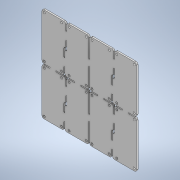
# Autodesk Inventor part: Part1
Saved by Autodesk Inventor 2021 (Build 250183000, 183)
## iProperties
Created: 2021-05-25
Part Number: Part1
Material: 一般
Document SubType Name: Modeling
Designer: admin
Density: 1 g/cm^3
Appearance: 既定
Author: admin
Autodesk Inventor part; units mm, degrees
ref_plane "YZ Plane" through (0, 0, 0) normal (1, 0, 0) x (0, 1, 0)
ref_plane "XZ Plane" through (0, 0, 0) normal (0, 1, 0) x (-1, 0, 0)
ref_plane "XY Plane" through (0, 0, 0) normal (0, 0, 1) x (1, 0, 0)
sketch "スケッチ1" plane through (0, 0, 0) normal (0, 0, 1) x (1, 0, 0)
  line L0 (0, 0) -> (49.5, 0)
  line L1 (49.5, 0) -> (49.5, 49.5)
  line L2 (49.5, 49.5) -> (0, 49.5)
  line L3 (0, 49.5) -> (0, 0)
  dimension "d0" = 49.5
  dimension "d1" = 49.5
  constraints: 8 end point, 2 parallel, 1 horizontal, 1 perpendicular
  measures "d0" distance of L2.end L1.end
  measures "d1" distance of L1.end L0.end
extrude "押し出し1" add sketch "スケッチ1" along normal blind 1.6
sketch "スケッチ2" plane through (0, 0, 1.6) normal (0, 0, 1) x (1, 0, 0)
  line L0 (0, 0) -> (49.5, 0) projected
  line L1 (24.75, 0) -> (24.75, 49.5) construction
  line L2 (49.5, 49.5) -> (0, 49.5) projected
  line L3 (49.5, 0) -> (49.5, 49.5) projected
  line L4 (49.5, 24.75) -> (0, 24.75) construction
  line L5 (0, 49.5) -> (0, 0) projected
  arc A0 (24.75, 23.25) -> (26.25, 24.75) centre (24.75, 24.75) ccw
  line L6 (26.25, 49.5) -> (26.25, 33.125) construction
  line L7 (23.25, 24.75) -> (23.25, 16.375)
  arc A1 (24.75, 26.25) -> (23.25, 24.75) centre (24.75, 24.75) ccw
  line L8 (24.75, 23.25) -> (24.25, 23.25)
  line L9 (24.75, 26.25) -> (25.25, 26.25)
  line L10 (24.25, 23.25) -> (24.25, 16.375)
  line L11 (25.25, 49.5) -> (25.25, 33.125) construction
  line L12 (23.25, 16.375) -> (24.25, 16.375)
  line L13 (24.25, 16.375) -> (24.25, 8.375) construction
  line L14 (24.25, 8.375) -> (23.25, 8.375) construction
  line L15 (23.25, 8.375) -> (23.25, 16.375) construction
  line L16 (25.25, 41.125) -> (26.25, 41.125) construction
  line L17 (26.25, 41.125) -> (26.25, 33.125) construction
  line L18 (26.25, 33.125) -> (25.25, 33.125)
  line L19 (25.25, 33.125) -> (25.25, 41.125) construction
  line L20 (21.3132, 37.125) -> (36.5279, 37.125) construction
  line L21 (13.313, 12.375) -> (31.136, 12.375) construction
  line L22 (23.25, 16.375) -> (23.25, 0) construction
  line L23 (24.25, 16.375) -> (24.25, 0.75) construction
  line L24 (25.25, 33.125) -> (25.25, 26.25)
  line L25 (26.25, 33.125) -> (26.25, 24.75)
  line L26 (25.25, 49.5) -> (26.25, 49.5)
  line L27 (26.25, 49.5) -> (26.25, 41.125)
  line L28 (26.25, 41.125) -> (25.25, 41.125)
  line L29 (25.25, 41.125) -> (25.25, 49.5)
  line L30 (23.25, 8.375) -> (24.25, 8.375)
  line L31 (24.25, 8.375) -> (24.25, 0)
  line L32 (24.25, 0) -> (23.25, 0)
  line L33 (23.25, 0) -> (23.25, 8.375)
  point P0 (25.25, 0)
  point P1 (25.25, 49.5)
  point P2 (25.25, 37.125)
  point P3 (24.25, 12.375)
  point P4 (25.25, 37.125)
  point P5 (24.25, 0)
  dimension "d31" = 3
  dimension "d32" = 1
  dimension "d33" = 8
  dimension "d34" = 24.75
  dimension "d35" = 49.5
  dimension "d36" = 12.375
  constraints: 60 end point, 16 parallel, 13 point on line, 10 perpendicular, 8 collinear, 8 tangent, 7 midpoint, 6 horizontal, 4 point on circle, 2 centre point, 2 vertical, 3 other
  measures "d31" diameter of A0
  measures "d32" distance between parallel lines of L10 L7
  measures "d33" distance between parallel lines of L16 L18
  measures "d34" distance between parallel lines of L0 L4
  measures "d35" distance between parallel lines of L2 L0
  measures "d36" distance between parallel lines of L20 L2
extrude "押し出し2" cut sketch "スケッチ2" against normal up to surface (1.6 mm away) contours L33 L30 L31 L0 | L2 L27 L28 L29 | L8 L10 L12 L7 A1 L9 L24 L18 L25 A0
sketch "スケッチ3" plane through (0, 0, 1.6) normal (0, 0, 1) x (1, 0, 0)
  line L0 (47, 2.5) -> (2.5, 2.5)
  line L1 (2.5, 2.5) -> (2.5, 47)
  line L2 (2.5, 47) -> (47, 47)
  line L3 (47, 47) -> (47, 2.5)
  line L4 (28.75, 2.5) -> (28.75, 47)
  line L5 (20.75, 2.5) -> (20.75, 47)
  line L6 (0, 0) -> (23.25, 0) projected
  line L7 (49.5, 0) -> (49.5, 49.5) projected
  line L8 (49.5, 24.75) -> (0, 24.75) construction
  line L9 (0, 49.5) -> (0, 0) projected
  line L10 (24.75, 2.2211) -> (24.75, 28.2211) construction
  line L11 (26.301, 18.5) -> (26.301, 29.5)
  line L12 (26.301, 10.6062) -> (26.301, 18.8408) construction
  line L13 (23.199, 11.5293) -> (23.199, 19.7639) construction
  line L14 (23.199, 29.0771) -> (23.199, 18.0771)
  line L15 (23.25, 0) -> (23.25, 8.375) projected
  point P0 (0.5, 0)
  point P1 (23.75, 0)
  point P2 (49.5, 0.5)
  point P3 (49.5, 47.5)
  point P4 (0, 47.5)
  point P5 (0, 0.5)
  point P6 (49, 0)
  point P7 (24.75, 24.75)
  dimension "d16" = 2.5
  dimension "d18" = 2.5
  dimension "d37" = 2.5
  constraints: 24 end point, 8 coincident, 5 point on line, 3 midpoint, 3 perpendicular, 2 collinear, 2 parallel, 2 vertical, 1 horizontal, 4 other
  measures "d16" distance between parallel lines of L0 L6
  measures "d18" distance between parallel lines of L9 L1
  measures "d37" distance between parallel lines of L5 L15
hole "穴1" at (47, 2.5, 1.6) at (28.75, 2.5, 1.6) at (20.75, 2.5, 1.6) at (2.5, 2.5, 1.6) at (2.5, 47, 1.6) at (20.75, 47, 1.6) at (28.75, 47, 1.6) at (47, 47, 1.6) direction (0, 0, -1) diameter 2.2 end through all
pattern_linear "矩形状パターン1" count 2 spacing 50.5 along (1, 0, 0) count 2 spacing 50.5 along (0, 1, 0)
sketch "スケッチ7" plane through (0, 0, 1.6) normal (0, 0, 1) x (1, 0, 0)
  line L0 (8.625, 50.5) -> (14.625, 50.5)
  line L1 (14.625, 50.5) -> (14.625, 49.5)
  line L2 (14.625, 49.5) -> (8.625, 49.5)
  line L3 (8.625, 49.5) -> (8.625, 50.5)
  line L4 (34.875, 50.5) -> (40.875, 50.5)
  line L5 (40.875, 50.5) -> (40.875, 49.5)
  line L6 (40.875, 49.5) -> (34.875, 49.5)
  line L7 (34.875, 49.5) -> (34.875, 50.5)
  line L8 (59.125, 50.5) -> (65.125, 50.5)
  line L9 (65.125, 50.5) -> (65.125, 49.5)
  line L10 (65.125, 49.5) -> (59.125, 49.5)
  line L11 (59.125, 49.5) -> (59.125, 50.5)
  line L12 (85.375, 50.5) -> (91.375, 50.5)
  line L13 (91.375, 50.5) -> (91.375, 49.5)
  line L14 (91.375, 49.5) -> (85.375, 49.5)
  line L15 (85.375, 49.5) -> (85.375, 50.5)
  line L16 (49.5, 72.25) -> (50.5, 72.25)
  line L17 (50.5, 72.25) -> (50.5, 78.25)
  line L18 (50.5, 78.25) -> (49.5, 78.25)
  line L19 (49.5, 78.25) -> (49.5, 72.25)
  line L20 (49.5, 27.75) -> (50.5, 27.75)
  line L21 (50.5, 27.75) -> (50.5, 21.75)
  line L22 (50.5, 21.75) -> (49.5, 21.75)
  line L23 (49.5, 21.75) -> (49.5, 27.75)
  line L24 (11.625, 50.5) -> (11.625, 49.5) construction
  line L25 (37.875, 50.5) -> (37.875, 49.5) construction
  line L26 (62.125, 50.5) -> (62.125, 49.5) construction
  line L27 (88.375, 50.5) -> (88.375, 49.5) construction
  line L28 (49.5, 24.75) -> (50.5, 24.75) construction
  line L29 (49.5, 75.25) -> (50.5, 75.25) construction
  line L30 (0, 50.5) -> (23.25, 50.5) projected
  line L31 (49.5, 49.5) -> (26.25, 49.5) projected
  line L32 (50.5, 50.5) -> (73.75, 50.5) projected
  line L33 (100, 49.5) -> (76.75, 49.5) projected
  line L34 (49.5, 50.5) -> (49.5, 100) projected
  line L35 (50.5, 49.5) -> (50.5, 0) projected
  point P0 (0, 0)
  point P1 (11.625, 50.5)
  dimension "d41" = 6
  constraints: 60 end point, 18 midpoint, 12 parallel, 10 point on line, 8 collinear, 6 horizontal, 6 perpendicular, 5 equal length
  measures "d41" distance between parallel lines of L16 L18
extrude "押し出し5" add sketch "スケッチ7" against normal up to surface (1.6 mm away)
fillet "フィレット3" radius 0.5 64 edges at (24.25, 8.375, 0.8) (23.25, 8.375, 0.8) (49.5, 21.75, 0.8) (50.5, 21.75, 0.8) (74.75, 8.375, 0.8) (73.75, 8.375, 0.8) (74.75, 16.375, 0.8) (73.75, 16.375, 0.8) (74.75, 23.25, 0.8) (75.75, 26.25, 0.8) (75.75, 33.125, 0.8) (76.75, 33.125, 0.8) (49.5, 27.75, 0.8) (50.5, 27.75, 0.8) (23.25, 16.375, 0.8) (24.25, 16.375, 0.8) (24.25, 23.25, 0.8) (25.25, 26.25, 0.8) (25.25, 33.125, 0.8) (26.25, 33.125, 0.8) (25.25, 41.125, 0.8) (26.25, 41.125, 0.8) (76.75, 41.125, 0.8) (75.75, 41.125, 0.8) (8.625, 49.5, 0.8) (8.625, 50.5, 0.8) (34.875, 49.5, 0.8) (59.125, 49.5, 0.8) (85.375, 49.5, 0.8) (85.375, 50.5, 0.8) (59.125, 50.5, 0.8) (34.875, 50.5, 0.8) (14.625, 50.5, 0.8) (40.875, 50.5, 0.8) (65.125, 50.5, 0.8) (91.375, 50.5, 0.8) (91.375, 49.5, 0.8) (65.125, 49.5, 0.8) (40.875, 49.5, 0.8) (14.625, 49.5, 0.8) (24.25, 58.875, 0.8) (50.5, 72.25, 0.8) (74.75, 58.875, 0.8) (73.75, 58.875, 0.8) (49.5, 72.25, 0.8) (23.25, 58.875, 0.8) (25.25, 83.625, 0.8) (25.25, 76.75, 0.8) (75.75, 76.75, 0.8) (75.75, 83.625, 0.8) (76.75, 83.625, 0.8) (26.25, 83.625, 0.8) (24.25, 73.75, 0.8) (74.75, 73.75, 0.8) (73.75, 66.875, 0.8) (74.75, 66.875, 0.8) (50.5, 78.25, 0.8) (49.5, 78.25, 0.8) (23.25, 66.875, 0.8) (24.25, 66.875, 0.8) (25.25, 91.625, 0.8) (26.25, 91.625, 0.8) (76.75, 91.625, 0.8) (75.75, 91.625, 0.8)
fillet "フィレット4" radius 2 32 edges at (100, 49.5, 0.8) (100, 50.5, 0.8) (76.75, 49.5, 0.8) (75.75, 49.5, 0.8) (73.75, 50.5, 0.8) (50.5, 49.5, 0.8) (49.5, 49.5, 0.8) (49.5, 50.5, 0.8) (26.25, 49.5, 0.8) (25.25, 49.5, 0.8) (23.25, 50.5, 0.8) (0, 49.5, 0.8) (0, 50.5, 0.8) (0, 0, 0.8) (24.25, 0, 0.8) (50.5, 0, 0.8) (74.75, 0, 0.8) (23.25, 0, 0.8) (49.5, 0, 0.8) (73.75, 0, 0.8) (100, 0, 0.8) (24.25, 50.5, 0.8) (50.5, 50.5, 0.8) (74.75, 50.5, 0.8) (100, 100, 0.8) (75.75, 100, 0.8) (49.5, 100, 0.8) (25.25, 100, 0.8) (0, 100, 0.8) (26.25, 100, 0.8) (50.5, 100, 0.8) (76.75, 100, 0.8)
equation "\"d18\" = d16"
